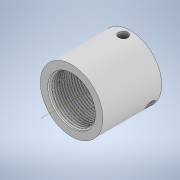
# Autodesk Inventor part: brakeStop
Saved by Autodesk Inventor 2021.1 (Build 251245000, 245)
## iProperties
Created: 2020-08-18
Part Number: brakeStop
Material: Generic
Document SubType Name: Modeling
Designer: robst
Density: 1 g/cm^3
Appearance: Default
Author: robst
Autodesk Inventor part; units mm, degrees
ref_plane "YZ Plane" through (0, 0, 0) normal (1, 0, 0) x (0, 1, 0)
ref_plane "XY Plane" through (0, 0, 0) normal (0, 0, 1) x (1, 0, 0)
sketch "Sketch3" plane through (0, 0, 0) normal (0, 0, 1) x (1, 0, 0)
  circle A0 centre (0, 0) radius 8.0645
  circle A1 centre (0, 0) radius 26.9875
  dimension "d8" = 16.129
  dimension "d9" = 53.975
  constraints: 2 centre point, 2 coincident
  measures "d8" diameter of A0
  measures "d9" diameter of A1
extrude "Extrusion3" add sketch "Sketch3" along normal blind 50.8
sketch "Sketch4" plane through (0, 0, 50.8) normal (0, 0, 1) x (1, 0, 0)
  circle A0 centre (0, 0) radius 20.6146
  dimension "d12" = 41.2293
  constraints: 1 centre point, 1 coincident
  measures "d12" diameter of A0
extrude "Extrusion4" cut sketch "Sketch4" against normal blind 38.1
sketch "Sketch5" plane through (0, 0, 0) normal (1, 0, 0) x (0, 1, 0)
  line L0 (20.6146, 50.8) -> (20.6146, 12.7) projected
  line L1 (26.9875, 50.8) -> (-26.9875, 50.8) projected
  line L2 (20.6146, 50.8) -> (20.6146, 50.8)
  line L3 (20.6146, 50.8) -> (19.4666, 50.1372)
  line L4 (19.4666, 49.75) -> (20.6146, 49.0872)
  arc A0 (19.4666, 50.1372) -> (19.4666, 49.75) centre (19.5783, 49.9436) ccw
  line L5 (0, -7.62) -> (0, 45.72) construction
  line L6 (20.6146, 49.0872) -> (20.6146, 50.8)
  point P0 (0, 0)
  dimension "d15" = 60
  dimension "d17" = 0.2235
  dimension "d18" = 19.3548
  dimension "d27" = 0
  constraints: 8 end point, 2 point on circle, 2 tangent, 1 centre point, 1 collinear, 1 equal length, 1 point on line, 1 vertical
  measures "d15" angle of L4 L3
  measures "d17" radius of A0
  measures "d18" distance edge to line of A0 L5
  measures "d27" distance of L2.end L0.start
coil "Coil2" sketch "Sketch5" operation add axis through (0, 0, -10) along (0, 0, -1) pitch 2.1167 turns 18 hand right
ref_plane "Work Plane1" through (0, 26.9875, 0) normal (0, 1, 0) x (-1, 0, 0)
sketch "Sketch6" plane through (0, 26.9875, 0) normal (0, 1, 0) x (-1, 0, 0)
  point P0 (0, 0)
  point P1 (0, 6.35)
  dimension "d37" = 6.35
  measures "d37" distance of point (0, 6.35) point (0, 0)
hole "Hole1" at (0, 26.9875, 6.35) direction (0, -1, 0) diameter 6.7564 depth 26.9875 counterbore diameter 8.0264 counterbore depth 7.3406
pattern_circular "Circular Pattern1" count 3 over 360 about axis through (0, 0, -10) along (0, 0, 1) of "Hole1"
equation "\"d8\" = innerDiameter"
equation "\"d9\" = outsideDiameter"
equation "\"d10\" = lengthOfBrakeStop"
equation "\"d12\" = majorDiameter"
equation "\"d13\" = depthOfThread"
equation "\"d17\" = rootRadius"
equation "\"d18\" = 0.5 * minorDiameter"
equation "\"d28\" = pitch"
equation "\"d29\" = depthOfThread"
equation "\"innerDiameter\" = 16.129"
equation "\"heightOfBrake\" = 6.35"
equation "\"majorDiameter\" = 41.22928"
equation "\"pitchDiameter\" = 39.85514"
equation "\"minorDiameter\" = 38.7096"
equation "\"crestFlat\" = 0.4318"
equation "\"rootRadius\" = 0.22352"
equation "\"threadDepth\" = 1.52146"
equation "\"outsideDiameter\" = 53.975"
equation "\"lengthOfBrakeStop\" = 50.8"
equation "\"depthOfThread\" = lengthOfBrakeStop - brakeStopLength"
equation "\"d36\" = 0.5 * outsideDiameter"
equation "\"brakeStopLength\" = 12.7"
equation "\"pitch\" = 2.116667"
body "Solid2"
